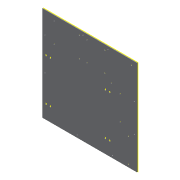
# Autodesk Inventor part: Power Board - Plate B2
Saved by Autodesk Inventor 2015 (Build 190159000, 159)
## iProperties
Created: 2015-01-11
Part Number: Power Board - Plate B2
Material: Generic
Document SubType Name: Sheet Metal
Designer: Peter
Density: 1 g/cm^3
Sheet Metal Rule: Default
Appearance: Default
Author: Peter
Autodesk Inventor part; units mm, degrees
ref_plane "YZ Plane" through (0, 0, 0) normal (1, 0, 0) x (0, 1, 0)
ref_plane "XZ Plane" through (0, 0, 0) normal (0, 1, 0) x (-1, 0, 0)
ref_plane "XY Plane" through (0, 0, 0) normal (0, 0, 1) x (1, 0, 0)
sketch "Sketch1" plane through (0, 0, 0) normal (0, 0, 1) x (1, 0, 0)
  line L0 (0, 0) -> (228.6, 0)
  line L1 (228.6, 0) -> (228.6, 228.6)
  line L2 (228.6, 228.6) -> (0, 228.6)
  line L3 (0, 228.6) -> (0, 0)
  dimension "d0" = 228.6
  dimension "d1" = 228.6
  measures "d0" distance of L2.end L1.end
  measures "d1" distance of L1.end L0.end
extrude "Plate1" add sketch "Sketch1" along normal blind 2.286
sketch "Sketch2" plane through (0, 0, 0) normal (0, 0, -1) x (-1, 0, 0)
  circle A0 centre (-28.5666, 168.1099) radius 1.8387 projected
  line L0 (-12.7161, 130.0825) -> (-12.7161, 139.643) projected
  line L1 (-12.7161, 130.0825) -> (-15.4564, 130.1971) projected
  line L2 (-15.4564, 130.1971) -> (-15.4564, 139.5284) projected
  line L3 (-12.7161, 139.643) -> (-15.4564, 139.5284) projected
  line L4 (-12.7161, 139.6958) -> (-12.7161, 130.0297) projected
  line L5 (-12.7161, 139.6958) -> (-15.4632, 139.5771) projected
  line L6 (-15.4632, 139.5771) -> (-15.4632, 130.1485) projected
  line L7 (-12.7161, 130.0297) -> (-15.4632, 130.1485) projected
  line L8 (-12.7161, 28.4825) -> (-12.7161, 38.043) projected
  line L9 (-12.7161, 28.4825) -> (-15.4564, 28.5971) projected
  line L10 (-15.4564, 28.5971) -> (-15.4564, 37.9284) projected
  line L11 (-12.7161, 38.043) -> (-15.4564, 37.9284) projected
  line L12 (-12.7161, 38.0958) -> (-12.7161, 28.4297) projected
  line L13 (-12.7161, 38.0958) -> (-15.4632, 37.9771) projected
  line L14 (-15.4632, 37.9771) -> (-15.4632, 28.5485) projected
  line L15 (-12.7161, 28.4297) -> (-15.4632, 28.5485) projected
  line L16 (-158.3812, 38.043) -> (-158.3812, 28.4825) projected
  line L17 (-158.3812, 38.043) -> (-155.6409, 37.9284) projected
  line L18 (-155.6409, 37.9284) -> (-155.6409, 28.5971) projected
  line L19 (-158.3812, 28.4825) -> (-155.6409, 28.5971) projected
  line L20 (-158.3812, 28.4297) -> (-158.3812, 38.0958) projected
  line L21 (-158.3812, 28.4297) -> (-155.6341, 28.5485) projected
  line L22 (-155.6341, 28.5485) -> (-155.6341, 37.9771) projected
  line L23 (-158.3812, 38.0958) -> (-155.6341, 37.9771) projected
  line L24 (-158.3812, 38.043) -> (-158.3812, 28.4825) projected
  line L25 (-158.3812, 38.043) -> (-155.6409, 37.9284) projected
  line L26 (-155.6409, 37.9284) -> (-155.6409, 28.5971) projected
  line L27 (-158.3812, 28.4825) -> (-155.6409, 28.5971) projected
  line L28 (-158.3812, 130.0297) -> (-158.3812, 139.6958) projected
  line L29 (-158.3812, 130.0297) -> (-155.6341, 130.1485) projected
  line L30 (-155.6341, 130.1485) -> (-155.6341, 139.5771) projected
  line L31 (-158.3812, 139.6958) -> (-155.6341, 139.5771) projected
  line L32 (-158.3812, 139.643) -> (-158.3812, 130.0825) projected
  line L33 (-158.3812, 139.643) -> (-155.6409, 139.5284) projected
  line L34 (-155.6409, 139.5284) -> (-155.6409, 130.1971) projected
  line L35 (-158.3812, 130.0825) -> (-155.6409, 130.1971) projected
  circle A1 centre (-207.805, 6.6) radius 2.5 projected
  circle A2 centre (-207.805, 65.3) radius 2.5 projected
  circle A3 centre (-187.575, 85.1796) radius 2.5 projected
  circle A4 centre (-187.575, 143.8796) radius 2.5 projected
  circle A5 centre (-215.4262, 217.5521) radius 2.1789 projected
  circle A6 centre (-166.4042, 155.8301) radius 2.1789 projected
  circle A7 centre (-150.622, 216.662) radius 1.905 projected
  circle A8 centre (-107.569, 216.662) radius 1.905 projected
  circle A9 centre (-107.569, 168.9124) radius 1.905 projected
  circle A10 centre (-150.622, 168.91) radius 1.905 projected
  circle A11 centre (-89.6028, 168.1099) radius 1.8387 projected
  circle A12 centre (-89.6028, 216.9541) radius 1.8387 projected
  circle A13 centre (-28.5666, 216.9541) radius 1.8387 projected
  circle A14 centre (-162.35, 134.8628) radius 2.3812
  circle A15 centre (-207.805, 6.6) radius 1.5875
  circle A16 centre (-207.805, 65.3) radius 1.5875
  circle A17 centre (-187.575, 85.1796) radius 1.5875
  circle A18 centre (-187.575, 143.8796) radius 1.5875
  circle A19 centre (-166.4042, 155.8301) radius 1.5875
  circle A20 centre (-150.622, 168.91) radius 1.5875
  circle A21 centre (-107.569, 168.9124) radius 1.5875
  circle A22 centre (-89.6028, 168.1099) radius 1.5875
  circle A23 centre (-28.5666, 168.1099) radius 1.5875
  circle A24 centre (-28.5666, 216.9541) radius 1.5875
  circle A25 centre (-89.6028, 216.9541) radius 1.5875
  circle A26 centre (-107.569, 216.662) radius 1.5875
  circle A27 centre (-150.622, 216.662) radius 1.5875
  circle A28 centre (-215.4262, 217.5521) radius 1.5875
  circle A29 centre (-151.8749, 134.8628) radius 2.3812
  line L36 (-155.6341, 37.9771) -> (-155.6409, 130.1971) construction
  line L37 (-15.4632, 37.9771) -> (-155.6341, 37.9771) construction
  line L38 (-155.6375, 84.0871) -> (-107.569, 84.0871) construction
  line L39 (-85.5487, 37.9771) -> (-85.5487, 82.6796) construction
  circle A30 centre (-162.35, 33.3114) radius 2.3812
  circle A31 centre (-151.8749, 33.3114) radius 2.3812
  circle A32 centre (-8.7473, 134.8628) radius 2.3812
  circle A33 centre (-19.2224, 134.8628) radius 2.3812
  circle A34 centre (-8.7473, 33.3114) radius 2.3812
  circle A35 centre (-19.2224, 33.3114) radius 2.3812
  dimension "d3" = 4.7625
  dimension "d4" = 3.9688
  dimension "x" = 3.175
  dimension "d6" = 3.175
  dimension "d7" = 3.175
  dimension "d8" = 3.175
  dimension "d9" = 3.175
  dimension "d10" = 3.175
  dimension "d11" = 3.175
  dimension "d12" = 3.175
  dimension "d13" = 3.175
  dimension "d14" = 3.175
  dimension "d15" = 3.175
  dimension "d16" = 3.175
  dimension "d17" = 3.175
  dimension "d18" = 3.175
  dimension "d19" = 4.7625
  dimension "d20" = 3.7592
  constraints: 22 centre point, 14 coincident, 8 end point, 6 symmetric about line, 2 horizontal, 2 midpoint, 1 vertical, 6 other
  measures "d3" diameter of A14
  measures "d4" horizontal distance of L28.end A14.centre
  measures "x" diameter of A15
  measures "d6" diameter of A16
  measures "d7" diameter of A17
  measures "d8" diameter of A18
  measures "d9" diameter of A19
  measures "d10" diameter of A20
  measures "d11" diameter of A21
  measures "d12" diameter of A22
  measures "d13" diameter of A23
  measures "d14" diameter of A24
  measures "d15" diameter of A25
  measures "d16" diameter of A26
  measures "d17" diameter of A27
  measures "d18" diameter of A28
  measures "d19" diameter of A29
  measures "d20" distance from line of L30 A29.centre
extrude "Cut1" cut sketch "Sketch2" against normal blind 2.286 contours A14 | A15 | A16 | A17 | A18 | A19 | A20 | A21 | A22 | A23 | A24 | A25 | A26 | A27 | A28 | A29 | A30 | A31 | A32 | A33 | A34 | A35
sketch "Sketch3" plane through (0, 0, 0) normal (0, 0, -1) x (-1, 0, 0)
  circle A0 centre (-187.575, 85.1796) radius 1.5875 projected
  circle A1 centre (-207.805, 6.6) radius 1.5875 projected
  circle A2 centre (-215.4262, 217.5521) radius 1.5875 projected
  circle A3 centre (-107.569, 168.9124) radius 1.5875 projected
  circle A4 centre (-150.622, 216.662) radius 1.5875 projected
  circle A5 centre (-89.6028, 216.9541) radius 1.5875 projected
  circle A6 centre (-28.5666, 168.1099) radius 1.5875 projected
  circle A7 centre (-8.7473, 134.8628) radius 2.3812 projected
  circle A8 centre (-19.2224, 33.3114) radius 2.3812 projected
  circle A9 centre (-162.35, 33.3114) radius 2.3812 projected
  circle A10 centre (-162.35, 134.8628) radius 2.3812 projected
  circle A11 centre (-151.8749, 134.8628) radius 2.3812 projected
  circle A12 centre (-151.8749, 33.3114) radius 2.3812 projected
  circle A13 centre (-8.7473, 33.3114) radius 2.3812 projected
  circle A14 centre (-19.2224, 134.8628) radius 2.3812 projected
  circle A15 centre (-89.6028, 168.1099) radius 1.5875 projected
  circle A16 centre (-28.5666, 216.9541) radius 1.5875 projected
  circle A17 centre (-107.569, 216.662) radius 1.5875 projected
  circle A18 centre (-150.622, 168.91) radius 1.5875 projected
  circle A19 centre (-166.4042, 155.8301) radius 1.5875 projected
  circle A20 centre (-207.805, 65.3) radius 1.5875 projected
  circle A21 centre (-187.575, 143.8796) radius 1.5875 projected
  line L0 (0, 0) -> (-228.6, 0) projected
  line L1 (0, 228.6) -> (0, 0) projected
  line L2 (-228.6, 228.6) -> (0, 228.6) projected
  line L3 (-228.6, 0) -> (-228.6, 228.6) projected
sketch "Sketch4" plane through (0, 0, 0) normal (0, 0, -1) x (-1, 0, 0)
  line L0 (0, 0) -> (-228.6, 0) projected
  line L1 (0, 228.6) -> (0, 0) construction
  line L2 (-228.6, 228.6) -> (0, 228.6) projected
  line L3 (-228.6, 0) -> (-228.6, 228.6) construction
  line L4 (-228.6, 228.6) -> (0, 228.6) projected
  line L5 (0, 222.25) -> (-228.6, 222.25) construction
  line L6 (-228.6, 228.6) -> (-228.6, 0) construction
  line L7 (0, 228.6) -> (-228.6, 228.6) construction
  line L8 (-222.25, 228.6) -> (-222.25, 0) construction
  line L9 (-228.6, 0) -> (0, 0) construction
  line L10 (-228.6, 6.35) -> (0, 6.35) construction
  line L11 (-6.35, 0) -> (-6.35, 228.6) construction
  circle A0 centre (-84.2642, 6.35) radius 1.5875
  circle A1 centre (-6.35, 97.3199) radius 1.5875
  circle A2 centre (-98.0716, 222.25) radius 1.5875
  point P0 (-169.4233, 6.35)
  point P1 (-222.25, 76.7211)
  point P2 (-222.25, 145.4671)
  point P3 (-158.2929, 222.25)
  point P4 (-6.35, 176.5259)
  dimension "d23" = 6.35
  dimension "d24" = 6.35
  dimension "d25" = 6.35
  dimension "d26" = 6.35
  dimension "d34" = 3.175
  dimension "d35" = 3.175
  dimension "d36" = 3.175
  constraints: 16 point on line, 8 end point, 4 perpendicular, 3 centre point, 3 coincident
  measures "d23" distance of L2.start L5.end
  measures "d24" distance of L1.start L11.end
  measures "d25" distance of L8.start L2.start
  measures "d26" distance of L0.end L10.start
  measures "d34" diameter of A0
  measures "d35" diameter of A1
  measures "d36" diameter of A2
hole "Hole1" at (6.35, 176.5259, 0) at (98.0716, 222.25, 0) at (158.2929, 222.25, 0) at (222.25, 145.4671, 0) at (222.25, 76.7211, 0) at (169.4233, 6.35, 0) direction (0, 0, 1) diameter 3.175 end through all
extrude "Cut2" cut sketch "Sketch4" against normal blind 2.286 contours A0
extrude "Cut3" cut sketch "Sketch4" against normal blind 2.286 contours A1
equation "\"d6\" = x"
equation "\"d7\" = x"
equation "\"d8\" = x"
equation "\"d9\" = x"
equation "\"d10\" = x"
equation "\"d11\" = x"
equation "\"d12\" = x"
equation "\"d13\" = x"
equation "\"d14\" = x"
equation "\"d15\" = x"
equation "\"d16\" = x"
equation "\"d17\" = x"
equation "\"d18\" = x"
equation "\"d21\" = Thickness"
equation "\"d32\" = Thickness"
equation "\"d37\" = Thickness"
equation "\"d39\" = Thickness"
equation "\"BendRadius\" = Thickness"
equation "\"BendReliefWidth\" = Thickness"
equation "\"BendReliefDepth\" = 0.5 * Thickness"
equation "\"CornerReliefSize\" = 4 * Thickness"
equation "\"MinimumRemnant\" = 2 * Thickness"
equation "\"TransitionRadius\" = BendRadius"
equation "\"JacobiRadiusSize\" = BendRadius"
equation "\"GapSize\" = Thickness"
equation "\"d2\" = BendRadius"
equation "\"Thickness\" = 2.286"
body "Solid1"
